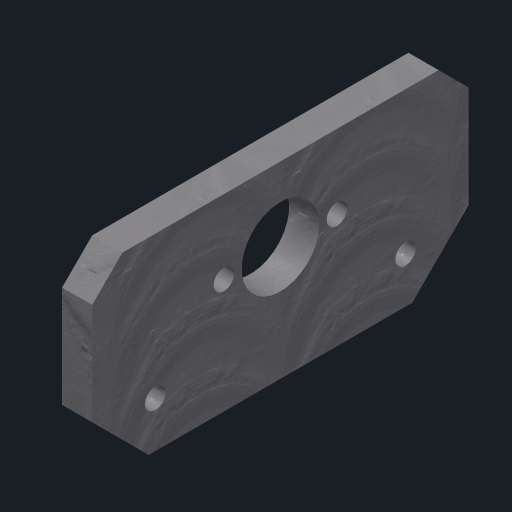
# Autodesk Inventor part: CAJA
Saved by Autodesk Inventor 2024.3 (Build 283343000, 343)
## iProperties
Created: 2024-06-29
Part Number: CAJA
Material: Steel, Mild, Welded
Document SubType Name: Modeling
Designer: Niler
Density: 7.85 g/cm^3
Appearance: Weld - Steel Mild
Author: Niler
Autodesk Inventor part; units mm, degrees
ref_plane "YZ Plane" through (0, 0, 0) normal (1, 0, 0) x (0, 1, 0)
ref_plane "XZ Plane" through (0, 0, 0) normal (0, 1, 0) x (-1, 0, 0)
ref_plane "XY Plane" through (0, 0, 0) normal (0, 0, 1) x (1, 0, 0)
sketch "Sketch1" plane through (0, 0, 0) normal (1, 0, 0) x (0, 1, 0)
  line L0 (-55, 110) -> (55, 110)
  line L1 (55, 110) -> (55, -110)
  line L2 (55, -110) -> (-55, -110)
  line L3 (-55, -110) -> (-55, 110)
  line L4 (-55, 110) -> (55, -110) construction
  line L5 (55, 110) -> (-55, -110) construction
  circle A0 centre (-15, 30) radius 4.1
  circle A1 centre (-15, -30) radius 4.1
  circle A2 centre (-15, 0) radius 5
  line L6 (-15, 30) -> (-15, -30) construction
  line L7 (48, -103) -> (48, 103)
  line L8 (48, 103) -> (-48, 103)
  line L9 (-48, 103) -> (-48, -103)
  line L10 (-48, -103) -> (48, -103)
  point P0 (0, 0)
  dimension "d0" = 60
  dimension "d1" = 8.2
  dimension "d2" = 220
  dimension "d3" = 110
  dimension "d4" = 7
  dimension "d35" = 10
  dimension "d36" = 15
  constraints: 22 end point, 4 parallel, 3 centre point, 3 midpoint, 2 perpendicular, 1 coincident, 1 equal radius, 1 horizontal, 1 horizontal alignment, 1 vertical alignment, 3 other
  measures "d0" distance of L6.end L6.start
  measures "d1" diameter of A0
  measures "d2" distance between parallel lines of L2 L0
  measures "d3" distance of L0.start L0.end
  measures "d4" distance between parallel lines of L1 L7
  measures "d35" diameter of A2
  measures "d36" distance of A2.centre point (0, 0)
extrude "Extrusion1" add sketch "Sketch1" along normal blind 8 contours L0 L1 L2 L3 | A0 | A1 | L10 L9 L8 L7
sketch "Sketch2" plane through (8, 0, 0) normal (1, 0, 0) x (0, 0, -1)
  line L0 (110, -55) -> (110, 55) projected
  line L1 (110, 55) -> (-110, 55) projected
  line L2 (-110, 55) -> (-110, -55) projected
  line L3 (-110, -55) -> (110, -55) projected
  line L4 (-33.234, -33.234) -> (33.234, -33.234) construction
  line L5 (33.234, -33.234) -> (33.234, 33.234) construction
  line L6 (33.234, 33.234) -> (-33.234, 33.234) construction
  line L7 (-33.234, 33.234) -> (-33.234, -33.234) construction
  line L8 (-33.234, -33.234) -> (33.234, 33.234) construction
  line L9 (33.234, -33.234) -> (-33.234, 33.234) construction
  circle A0 centre (0, 0) radius 47 construction
  circle A1 centre (33.234, 33.234) radius 2.75
  circle A2 centre (-33.234, 33.234) radius 2.75
  circle A3 centre (0, 0) radius 47 construction
  circle A4 centre (-33.234, -33.234) radius 2.75
  circle A5 centre (0, 0) radius 47 construction
  circle A6 centre (33.234, -33.234) radius 2.75
  circle A7 centre (0, 0) radius 47 construction
  point P0 (0, 0)
  point P1 (0, 0)
  dimension "d12" = 94
  dimension "d13" = 5.5
  dimension "d16" = 360
  constraints: 12 end point, 7 coincident, 4 centre point, 2 parallel, 2 perpendicular, 1 horizontal, 1 midpoint, 31 other
  measures "d13" diameter of A1
extrude "Extrusion3" cut sketch "Sketch2" against normal through all contours A1 | A2 | A4 | A6
sketch "Sketch3" plane through (0, 0, 0) normal (-1, 0, 0) x (0, 0, 1)
  circle A0 centre (33.234, -33.234) radius 2.75 projected
  circle A1 centre (33.234, 33.234) radius 2.75 projected
  circle A2 centre (-33.234, -33.234) radius 2.75 projected
  circle A3 centre (-33.234, 33.234) radius 2.75 projected
  circle A4 centre (0, -15) radius 5 projected
  circle A5 centre (-33.234, 33.234) radius 4.5
  circle A6 centre (33.234, 33.234) radius 2.75 projected
  circle A7 centre (33.234, 33.234) radius 4.5
  circle A8 centre (-33.234, -33.234) radius 4.5
  circle A9 centre (33.234, -33.234) radius 4.5
  point P0 (0, 0)
  dimension "d20" = 9
  constraints: 4 centre point, 4 coincident, 3 equal radius
  measures "d20" diameter of A5
extrude "Extrusion4" cut sketch "Sketch3" against normal blind 3 contours A0 | A1 | A2 | A3 | A5 | A7 | A8 | A9
sketch "Sketch4" plane through (8, 0, 0) normal (1, 0, 0) x (0, 0, -1)
  circle A0 centre (-33.234, -33.234) radius 2.75 projected
  circle A1 centre (-33.234, 33.234) radius 2.75 projected
  circle A2 centre (33.234, -33.234) radius 2.75 projected
  circle A3 centre (33.234, 33.234) radius 2.75 projected
  line L0 (110, -55) -> (110, 55) projected
  line L1 (110, 55) -> (-110, 55) projected
  line L2 (-110, 55) -> (-110, -55) projected
  line L3 (-110, -55) -> (110, -55) projected
  circle A4 centre (0, -15) radius 5 projected
  circle A5 centre (0, -15) radius 10.3
  point P0 (0, 0)
  dimension "d24" = 20.6
  constraints: 1 centre point, 1 coincident
  measures "d24" diameter of A5
extrude "Extrusion5" cut sketch "Sketch4" against normal through all contours A4 | A5
sketch "Sketch7" plane through (0, 0, 0) normal (-1, 0, 0) x (0, 0, 1)
  line L0 (-50, -45.3941) -> (50, -45.3941)
  line L1 (50, -45.3941) -> (50, 4.6059)
  line L2 (50, 4.6059) -> (-50, 4.6059)
  line L3 (-50, 4.6059) -> (-50, -45.3941)
  circle A0 centre (-30, -15) radius 4.1 projected
  circle A1 centre (30, -15) radius 4.1 projected
  line L4 (-110, -55) -> (-110, 55) projected
  line L5 (-110, 55) -> (110, 55) projected
  line L6 (110, 55) -> (110, -55) projected
  line L7 (110, -55) -> (-110, -55) projected
  point P0 (0, 4.6059)
  point P1 (0, 4.6059)
  point P2 (0, -15)
  dimension "d37" = 50
  dimension "d38" = 100
  constraints: 8 end point, 2 parallel, 1 coincident, 1 horizontal, 1 midpoint, 1 perpendicular, 1 vertical alignment
  measures "d37" distance of L2.end L0.start
  measures "d38" distance between parallel lines of L1 L3
extrude "Extrusion8" cut sketch "Sketch7" against normal through all
chamfer "Chamfer3" distance 15 angle 45 2 edges at (4, -45.3941, -50) (4, -45.3941, 50)
chamfer "Chamfer4" distance 8 angle 45 2 edges at (4, 4.6059, -50) (4, 4.6059, 50)
sketch "Sketch8" plane through (0, 0, 0) normal (-1, 0, 0) x (0, 0, 1)
  circle A0 centre (-30, -15) radius 4.1 projected
  circle A1 centre (30, -15) radius 4.1 projected
  circle A2 centre (-30, -15) radius 6
  circle A3 centre (30, -15) radius 6
  point P0 (0, 0)
  dimension "d47" = 12
  constraints: 2 centre point, 2 coincident, 1 equal radius
  measures "d47" diameter of A2
extrude "Extrusion9" add sketch "Sketch8" along normal blind 5
sketch "Sketch9" plane through (8, 0, 0) normal (1, 0, 0) x (0, 0, -1)
  circle A0 centre (-30, -15) radius 4.1 projected
  circle A1 centre (30, -15) radius 4.1 projected
  point P0 (0, 0)
extrude "Extrusion10" add sketch "Sketch9" against normal blind 4
sketch "Sketch10" plane through (0, 0, 0) normal (-1, 0, 0) x (0, 0, 1)
  circle A0 centre (0, -15) radius 10.3 projected
  circle A1 centre (-15, -15) radius 2.75
  circle A2 centre (15, -15) radius 2.75
  line L0 (-15, -15) -> (15, -15) construction
  point P0 (0, 0)
  dimension "d52" = 30
  dimension "d53" = 5.5
  constraints: 2 centre point, 2 end point, 1 coincident, 1 equal radius, 1 horizontal, 1 midpoint
  measures "d52" distance of L0.end L0.start
  measures "d53" diameter of A1
extrude "Extrusion11" cut sketch "Sketch10" against normal through all contours A1 | A2
fillet "Fillet2" radius 2 2 edges at (0, -15, -36) (0, -15, 24)
body "Solid1"
